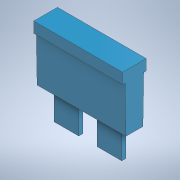
# Autodesk Inventor part: fuse
Saved by Autodesk Inventor 2021.5 (Build 255421000, 421)
## iProperties
Created: 2025-01-02
Part Number: fuse
Material: Generic
Document SubType Name: Modeling
Designer: email
Density: 1 g/cm^3
Appearance: Default
Author: email
Autodesk Inventor part; units mm, degrees
ref_plane "YZ Plane" through (0, 0, 0) normal (1, 0, 0) x (0, 1, 0)
ref_plane "XZ Plane" through (0, 0, 0) normal (0, 1, 0) x (-1, 0, 0)
ref_plane "XY Plane" through (0, 0, 0) normal (0, 0, 1) x (1, 0, 0)
sketch "Sketch1" plane through (0, 0, 0) normal (0, 1, 0) x (-1, 0, 0)
  line L0 (0, 0) -> (19.1, 0)
  line L1 (19.1, 0) -> (19.1, -5.1)
  line L2 (19.1, -5.1) -> (0, -5.1)
  line L3 (0, -5.1) -> (0, 0)
  dimension "d0" = 19.1
  dimension "d1" = 5.1
  constraints: 8 end point, 2 parallel, 1 horizontal, 1 perpendicular
  measures "d0" distance of L1.end L2.end
  measures "d1" distance of L0.end L1.end
extrude "Extrusion1" add sketch "Sketch1" against normal blind 2.29
sketch "Sketch2" plane through (0, 0, 0) normal (1, 0, 0) x (0, 1, 0)
  line L0 (-2.29, -5.1) -> (-2.29, 0) projected
  line L1 (-2.29, -4.375) -> (-12.29, -4.375) construction
  line L2 (-12.29, -4.375) -> (-12.29, -0.725)
  line L3 (-12.29, -0.725) -> (-2.29, -0.725) construction
  line L4 (-2.29, -0.725) -> (-2.29, -4.375)
  line L5 (0, -5.1) -> (-2.29, -5.1) projected
  line L6 (-2.29, -4.55) -> (-2.29, -0.55)
  line L7 (-2.29, -4.55) -> (-12.29, -4.375)
  line L8 (-2.29, -0.55) -> (-12.29, -0.725)
  point P0 (0, 0)
  dimension "d5" = 3.65
  dimension "d6" = 0.725
  dimension "d7" = 4
  dimension "d8" = 0.55
  dimension "d19" = 10
  constraints: 14 end point, 3 point on line, 2 parallel, 1 horizontal, 1 perpendicular
  measures "d5" distance of L1.end L2.end
  measures "d6" distance between parallel lines of L5 L1
  measures "d7" distance of L6.start L6.end
  measures "d8" distance from line of L5 L6.start
  measures "d19" distance between parallel lines of L0 L2
extrude "Extrusion2" add sketch "Sketch2" against normal blind 19.1
sketch "Sketch3" plane through (0, -12.29, -4.375) normal (0, -1, 0) x (1, 0, 0)
  line L0 (-16.8, 2.25) -> (-2.3, 2.25) construction
  line L1 (-2.3, 2.25) -> (-2.3, 1.4) construction
  line L2 (-2.3, 1.4) -> (-16.8, 1.4) construction
  line L3 (-16.8, 1.4) -> (-16.8, 2.25) construction
  line L4 (-19.1, 0) -> (-19.1, 3.65) projected
  line L5 (0, 3.65) -> (-19.1, 3.65) projected
  line L6 (-16.8, 2.25) -> (-11.55, 2.25)
  line L7 (-11.55, 2.25) -> (-11.55, 1.4)
  line L8 (-11.55, 1.4) -> (-16.8, 1.4)
  line L9 (-16.8, 1.4) -> (-16.8, 2.25)
  line L10 (-2.3, 2.25) -> (-7.55, 2.25)
  line L11 (-7.55, 2.25) -> (-7.55, 1.4)
  line L12 (-7.55, 1.4) -> (-2.3, 1.4)
  line L13 (-2.3, 1.4) -> (-2.3, 2.25)
  point P0 (0, 4.375)
  dimension "d11" = 14.5
  dimension "d12" = 2.3
  dimension "d13" = 0.85
  dimension "d14" = 1.4
  dimension "d15" = 5.25
  dimension "d16" = 5.25
  constraints: 24 end point, 6 parallel, 3 horizontal, 3 perpendicular, 2 point on line
  measures "d11" distance of L0.start L0.end
  measures "d12" distance between parallel lines of L4 L3
  measures "d13" distance of L2.end L0.start
  measures "d14" distance between parallel lines of L5 L0
  measures "d15" distance between parallel lines of L7 L3
  measures "d16" distance between parallel lines of L13 L11
extrude "Extrusion3" add sketch "Sketch3" along normal blind 6.42
body "Solid1"
